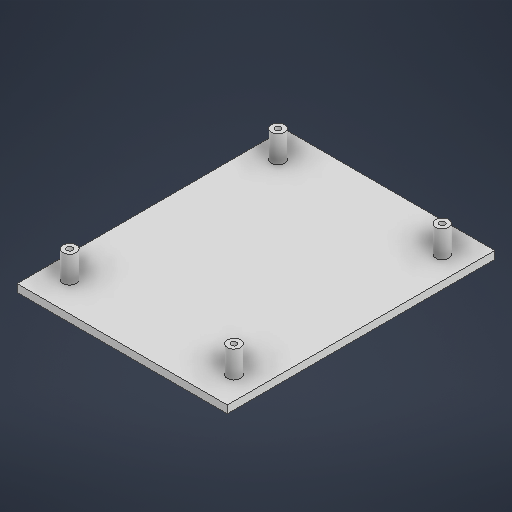
# Autodesk Inventor part: Base
Saved by Autodesk Inventor 2026 (Build 300175000, 175)
## iProperties
Created: 2026-02-15
Part Number: Base
Material: Generisch
Document SubType Name: Modeling
Designer: Jakob Dorninger
Density: 1 g/cm^3
Appearance: Vorgabe
Author: Jakob Dorninger
Autodesk Inventor part; units mm, degrees
ref_plane "YZ Plane" through (0, 0, 0) normal (1, 0, 0) x (0, 1, 0)
ref_plane "XZ Plane" through (0, 0, 0) normal (0, 1, 0) x (-1, 0, 0)
ref_plane "XY Plane" through (0, 0, 0) normal (0, 0, 1) x (1, 0, 0)
sketch "Skizze1" plane through (0, 0, 0) normal (0, 0, 1) x (1, 0, 0)
  line L0 (27.5, -35) -> (-27.5, -35)
  line L1 (-27.5, -35) -> (-27.5, 35)
  line L2 (-27.5, 35) -> (27.5, 35)
  line L3 (27.5, 35) -> (27.5, -35)
  line L4 (27.5, -35) -> (-27.5, 35) construction
  line L5 (-27.5, -35) -> (27.5, 35) construction
  point P0 (0, 0)
  dimension "d0" = 55
  dimension "d1" = 70
  constraints: 12 end point, 2 midpoint, 2 parallel, 1 horizontal, 1 perpendicular
  measures "d0" distance of L1.end L2.end
  measures "d1" distance of L0.end L1.end
extrude "Extrusion1" add sketch "Skizze1" along normal blind 2
sketch "Skizze2" plane through (0, 0, 2) normal (0, 0, 1) x (1, 0, 0)
  circle A0 centre (-21.5, 27.25) radius 1.75
  line L0 (0, -49) -> (0, 49) projected
  line L1 (-38.5, 0) -> (38.5, 0) projected
  circle A1 centre (-21.5, -27.25) radius 1.75
  circle A2 centre (21.5, 27.25) radius 1.75
  circle A3 centre (21.5, -27.25) radius 1.75
  point P0 (0, 0)
  dimension "d4" = 3.5
  dimension "d5" = 21.5
  dimension "d6" = 27.25
  dimension "d9" = 54.5
  dimension "d12" = 43
  constraints: 4 centre point, 1 horizontal, 1 vertical, 6 other
  measures "d4" diameter of A0
  measures "d5" horizontal distance of point (0, 0) A0.centre
  measures "d6" vertical distance of point (0, 0) A0.centre
  measures "d9" distance of A0.centre A1.centre
  measures "d12" distance of A0.centre A2.centre
extrude "Extrusion2" add sketch "Skizze2" along normal blind 7
sketch "Skizze3" plane through (-21.5, 27.25, 9) normal (0, 0, 1) x (1, 0, 0)
  circle A0 centre (0, 0) radius 1.75 projected
  line L0 (-17, -27.25) -> (60, -27.25) projected
  line L1 (21.5, -76.25) -> (21.5, 21.75) projected
  point P0 (21.5, -27.25)
  point P1 (0, -54.5)
  point P2 (43, 0)
  point P3 (43, -54.5)
  dimension "d19" = 54.5
  dimension "d22" = 43
  constraints: 1 coincident, 1 horizontal, 1 vertical, 3 other
  measures "d19" distance of point (0, 0) point (0, -54.5)
  measures "d22" distance of point (0, 0) point (43, 0)
hole "Bohrung1" at (-21.5, 27.25, 9) at (-21.5, -27.25, 9) at (21.5, 27.25, 9) at (21.5, -27.25, 9) direction (0, 0, -1) diameter 1.5 depth 7 tip angle 118
